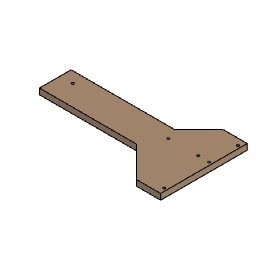
Brace TR (Autodesk Fusion 360 design; units mm, degrees)
Autodesk Fusion 360 part; units mm, degrees
sketch "Top" plane through (0, 0, 0) normal (0, 0, 1) x (1, 0, 0)
  line L0 (145, 175) -> (220, 175)
  line L1 (220, 175) -> (220, -93)
  line L2 (220, -93) -> (145, -93)
  line L3 (-250, 2) -> (-250, 100)
  line L4 (145, 175) -> (70, 100)
  line L5 (145, -93) -> (50, 2)
  line L6 (70, 100) -> (-250, 100)
  line L7 (50, 2) -> (-250, 2)
  line L8 (211, 175) -> (211, -93) construction
  line L9 (220, 66) -> (-250, 66) construction
  circle A0 centre (211, 66) radius 3.5
  circle A1 centre (211, 155) radius 3.5
  circle A2 centre (211, -73) radius 3.5
  circle A3 centre (85, 66) radius 3.5
  circle A4 centre (-211, 66) radius 3.5
  circle A5 centre (177, 66) radius 3.5
  dimension "d3" = 75
  dimension "d4" = 75
  dimension "d5" = 95
  dimension "d6" = 95
  dimension "d7" = 268
  dimension "d8" = 470
  dimension "d9" = 75
  dimension "d10" = 9
  dimension "d11" = 34
  dimension "d12" = 7
  dimension "d13" = 7
  dimension "d14" = 7
  dimension "d15" = 89
  dimension "d16" = 139
  dimension "d17" = 7
  dimension "d18" = 7
  dimension "d19" = 7
  dimension "d20" = 34
  dimension "d21" = 92
  dimension "d22" = 296
  constraint horizontal L0
  constraint vertical L1
  constraint horizontal L2
  constraint vertical L3
  constraint perpendicular L3 L6
  constraint perpendicular L3 L7
  constraint equal L0 L2
  constraint coincident L0 L8.start
  constraint coincident L2 L8.end
  constraint perpendicular L2 L8
  constraint coincident L1 L9.start
  constraint coincident L3 L9.end
  constraint perpendicular L3 L9
  constraint coincident L8 A0.centre
  constraint coincident L9 A0.centre
  constraint coincident L8 A1.centre
  constraint coincident L8 A2.centre
  constraint coincident L9 A3.centre
  constraint coincident L9 A4.centre
  constraint coincident L9 A5.centre
  measures "d3" horizontal distance of L0.start L4.end
  measures "d4" vertical distance of L0.start L4.end
  measures "d5" horizontal distance of L2.end L5.end
  measures "d6" vertical distance of L2.end L5.end
  measures "d7" distance of L0.end L1.end
  measures "d8" distance of L1 L3
  measures "d9" distance of L0.end L0.start
  measures "d10" distance of L1 L8
  measures "d11" distance of L6 L9
  measures "d12" diameter of A0
  measures "d13" diameter of A1
  measures "d14" diameter of A2
  measures "d15" distance of A0.centre A1.centre
  measures "d16" distance of A0.centre A2.centre
  measures "d17" diameter of A3
  measures "d18" diameter of A4
  measures "d19" diameter of A5
  measures "d20" distance of A0.centre A5.centre
  measures "d21" distance of A3.centre A5.centre
  measures "d22" distance of A3.centre A4.centre
extrude "Extrude1" add sketch "Top" along normal blind 18
named bodies: "Brace TR"
